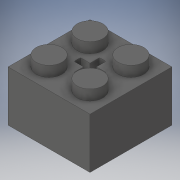
# Autodesk Inventor part: 2x2 tall things sticking out
Saved by Autodesk Inventor 2017 (Build 210142000, 142)
## iProperties
Created: 2018-05-17
Part Number: 2x2 tall things sticking out
Material: ABS Plastic
Document SubType Name: Modeling
Designer: Kyle
Density: 1.06 g/cm^3
Appearance: Gray
Author: Kyle
Autodesk Inventor part; units mm, degrees
ref_plane "YZ Plane" through (0, 0, 0) normal (1, 0, 0) x (0, 1, 0)
ref_plane "XZ Plane" through (0, 0, 0) normal (0, 1, 0) x (-1, 0, 0)
ref_plane "XY Plane" through (0, 0, 0) normal (0, 0, 1) x (1, 0, 0)
sketch "Sketch1" plane through (0, 0, 0) normal (0, 1, 0) x (-1, 0, 0)
  line L0 (0, 0) -> (15.5956, 0)
  line L1 (15.5956, 0) -> (15.5956, -15.5956)
  line L2 (15.5956, -15.5956) -> (0, -15.5956)
  line L3 (0, -15.5956) -> (0, 0)
  dimension "d0" = 15.5956
  dimension "d8" = 15.5956
  constraints: 8 end point, 2 parallel, 1 horizontal, 1 perpendicular
  measures "d0" distance of L1.end L2.end
  measures "d8" distance of L0.end L1.end
extrude "Extrusion1" add sketch "Sketch1" along normal blind 9.6088
sketch "Sketch2" plane through (0, 9.6088, 0) normal (0, 1, 0) x (1, 0, 0)
  line L0 (0, 0) -> (-3.8989, 0) construction
  line L1 (-3.8989, 0) -> (-3.8989, 3.8989) construction
  line L2 (-3.8989, 3.8989) -> (0, 3.8989) construction
  line L3 (0, 3.8989) -> (0, 0) construction
  circle A0 centre (-3.8989, 3.8989) radius 2.4498
  dimension "d11" = 3.8989
  dimension "d12" = 3.8989
  dimension "d13" = 4.8997
  constraints: 8 end point, 2 parallel, 1 centre point, 1 coincident, 1 horizontal, 1 perpendicular
  measures "d11" distance of L1.end L2.end
  measures "d12" distance of L0.end L1.end
  measures "d13" diameter of A0
extrude "Extrusion2" add sketch "Sketch2" along normal blind 1.9837
pattern_linear "Rectangular Pattern1" count 2 spacing 7.7978 along (0, 0, -1) count 2 spacing 7.7978 along (-1, 0, 0) of "Extrusion2"
shell "Shell1" thickness 1.4732 removed faces 1 at (-5.1985, 0, -5.1985)
sketch "Sketch3" plane through (-14.1224, 8.1356, -1.4732) normal (0, -1, 0) x (1, 0, 0)
  circle A0 centre (2.4257, -2.4257) radius 2.4498 construction
  circle A1 centre (10.2235, -10.2235) radius 2.4498 construction
  line L0 (2.4257, -2.4257) -> (10.2235, -10.2235) construction
  circle A2 centre (6.3246, -6.3246) radius 3.064
  circle A3 centre (6.3246, -6.3246) radius 2.4498
  point P0 (14.1224, 1.4732)
  dimension "d23" = 4.8997
  constraints: 2 centre point, 2 end point, 1 coincident, 1 midpoint
  measures "d23" diameter of A3
extrude "Extrusion3" add sketch "Sketch3" along normal up to surface (8.1356 mm away)
sketch "Sketch4" plane through (0, 9.6088, 0) normal (0, 1, 0) x (1, 0, 0)
  circle A0 centre (-7.7978, 7.7978) radius 2.4498 construction
  circle A1 centre (-7.7978, 7.7978) radius 2.4498 construction
  line L0 (-8.4103, 5.4258) -> (-7.1853, 5.4258) construction
  line L1 (-7.1853, 5.4258) -> (-7.1853, 10.1698) construction
  line L2 (-7.1853, 10.1698) -> (-8.4103, 10.1698) construction
  line L3 (-8.4103, 10.1698) -> (-8.4103, 5.4258) construction
  line L4 (-8.4103, 5.4258) -> (-7.1853, 10.1698) construction
  line L5 (-7.1853, 5.4258) -> (-8.4103, 10.1698) construction
  line L6 (-10.1698, 8.4103) -> (-5.4258, 8.4103) construction
  line L7 (-5.4258, 8.4103) -> (-5.4258, 7.1853) construction
  line L8 (-5.4258, 7.1853) -> (-10.1698, 7.1853) construction
  line L9 (-10.1698, 7.1853) -> (-10.1698, 8.4103) construction
  line L10 (-10.1698, 8.4103) -> (-5.4258, 7.1853) construction
  line L11 (-5.4258, 8.4103) -> (-10.1698, 7.1853) construction
  line L12 (-8.4103, 8.4103) -> (-8.4103, 10.1698)
  line L13 (-7.1853, 10.1698) -> (-7.1853, 8.4103)
  line L14 (-7.1853, 8.4103) -> (-5.4258, 8.4103)
  line L15 (-5.4258, 7.1853) -> (-7.1853, 7.1853)
  line L16 (-7.1853, 7.1853) -> (-7.1853, 5.4258)
  line L17 (-8.4103, 5.4258) -> (-8.4103, 7.1853)
  line L18 (-8.4103, 7.1853) -> (-10.1698, 7.1853)
  line L19 (-10.1698, 8.4103) -> (-8.4103, 8.4103)
  arc A2 (-10.1698, 8.4103) -> (-10.1698, 7.1853) centre (-7.7978, 7.7978) ccw
  arc A3 (-7.1853, 10.1698) -> (-8.4103, 10.1698) centre (-7.7978, 7.7978) ccw
  arc A4 (-5.4258, 7.1853) -> (-5.4258, 8.4103) centre (-7.7978, 7.7978) ccw
  arc A5 (-8.4103, 5.4258) -> (-7.1853, 5.4258) centre (-7.7978, 7.7978) ccw
  point P0 (0, 0)
  dimension "d26" = 1.2249
  dimension "d27" = 1.2249
  constraints: 40 end point, 10 point on circle, 8 point on line, 4 centre point, 4 midpoint, 4 parallel, 4 perpendicular, 3 collinear, 2 horizontal
  measures "d26" distance of L2.end L1.end
  measures "d27" distance of L6.end L7.end
extrude "Extrusion4" cut sketch "Sketch4" against normal through all
equation "\"d0\" = 2 * d1"
equation "\"d8\" = 2 * d1"
equation "\"d9\" = d3"
equation "\"d11\" = 0.5 * d1"
equation "\"d12\" = 0.5 * d1"
equation "\"d13\" = d4"
equation "\"d14\" = d5"
equation "\"d18\" = d1"
equation "\"d21\" = d1"
equation "\"d22\" = d6"
equation "\"d23\" = d4"
equation "\"d24\" = d5"
equation "\"d26\" = 0.25 * d4"
equation "\"d27\" = 0.25 * d4"
equation "\"d28\" = d5"
equation "\"d1\" = 7.7978"
equation "\"d2\" = 3.23596"
equation "\"d3\" = 9.60882"
equation "\"d4\" = 4.89966"
equation "\"d5\" = 1.98374"
equation "\"d6\" = 1.4732"
equation "\"d7\" = 1.23952"
body "Solid1"
